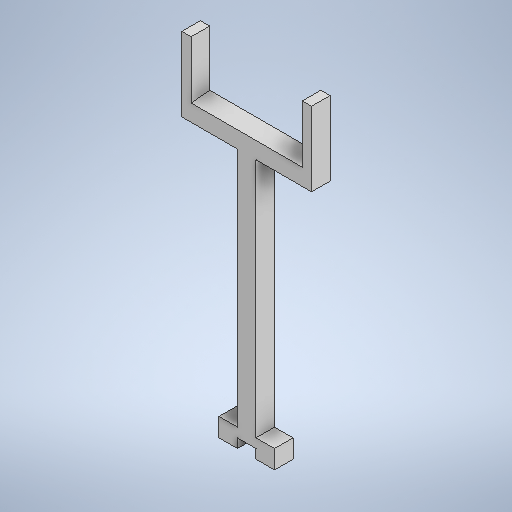
# Autodesk Inventor part: Sorting Holder x1
Saved by Autodesk Inventor 2025.3 (Build 293356000, 356)
## iProperties
Created: 2026-04-18
Part Number: Sorting Holder x1
Material: Generic
Document SubType Name: Modeling
Designer: kamal
Density: 1 g/cm^3
Appearance: Default
Author: kamal
Autodesk Inventor part; units mm, degrees
ref_plane "YZ Plane" through (0, 0, 0) normal (1, 0, 0) x (0, 1, 0)
ref_plane "XZ Plane" through (0, 0, 0) normal (0, 1, 0) x (-1, 0, 0)
sketch "Sketch2" plane through (0, 0, 0) normal (0, 0, 1) x (1, 0, 0)
  line L0 (0, 0) -> (0, 50) construction
  line L1 (0, 0) -> (0, 5)
  line L2 (0, 5) -> (-5, 5)
  line L3 (-5, 5) -> (-5, 0)
  line L4 (-5, 0) -> (-15, 0)
  line L5 (-15, 0) -> (-15, 5)
  line L6 (-15, 5) -> (-15, 10)
  line L7 (-15, 10) -> (-5, 10)
  line L8 (-5, 10) -> (-5, 140)
  line L9 (-5, 140) -> (-35, 140)
  line L10 (-35, 140) -> (-35, 180)
  line L11 (-35, 180) -> (-30, 180)
  line L12 (-30, 180) -> (-30, 150)
  line L13 (-30, 150) -> (0, 150)
  line L14 (0, 5) -> (5, 5)
  line L15 (5, 5) -> (5, 0)
  line L16 (15, 0) -> (15, 5)
  line L17 (15, 5) -> (15, 10)
  line L18 (15, 10) -> (5, 10)
  line L19 (5, 10) -> (5, 140)
  line L20 (5, 140) -> (35, 140)
  line L21 (35, 140) -> (35, 180)
  line L22 (35, 180) -> (30, 180)
  line L23 (30, 180) -> (30, 150)
  line L24 (30, 150) -> (0, 150)
  line L25 (5, 0) -> (15, 0)
  dimension "d6" = 50
  dimension "d7" = 5
  dimension "d8" = 5
  dimension "d9" = 10
  dimension "d10" = 130
  dimension "d11" = 30
  dimension "d12" = 40
  dimension "d13" = 5
  dimension "d14" = 30
  dimension "d21" = 5
  dimension "d22" = 5
  dimension "d24" = 0
  constraints: 52 end point, 11 symmetric about line, 8 perpendicular, 3 point on line, 3 vertical, 2 equal length, 2 horizontal
  measures "d6" distance of L0.start L0.end
  measures "d7" distance of L0.start L1.end
  measures "d8" distance of L1.end L2.end
  measures "d9" distance of L3.end L4.end
  measures "d10" distance of L7.end L8.end
  measures "d11" distance of L8.end L9.end
  measures "d12" distance of L9.end L10.end
  measures "d13" distance of L10.end L11.end
  measures "d14" distance of L11.end L12.end
  measures "d21" distance of L4.end L5.end
  measures "d22" distance of L2.end L3.end
  measures "d24" distance from line of L13.end L0
extrude "Extrusion1" add sketch "Sketch2" along normal mid plane 10
ref_plane "Work Plane1" through (0, 150, 5) normal (1, 0, 0) x (0, 0, -1)
sketch "Sketch3" plane through (0, 150, 5) normal (1, 0, 0) x (0, 0, -1)
  line L0 (0, 0) -> (10, 0)
  line L1 (0, 0) -> (0, -1)
  line L2 (10, -10) -> (0, -10) projected
  line L3 (0, -1) -> (10, 0)
  point P0 (5, -150)
  dimension "d27" = 1
  constraints: 6 end point, 1 horizontal, 1 perpendicular
  measures "d27" distance of L0.start L1.end
extrude "Extrusion2" cut sketch "Sketch3" along normal mid plane 60
body "Solid1"
